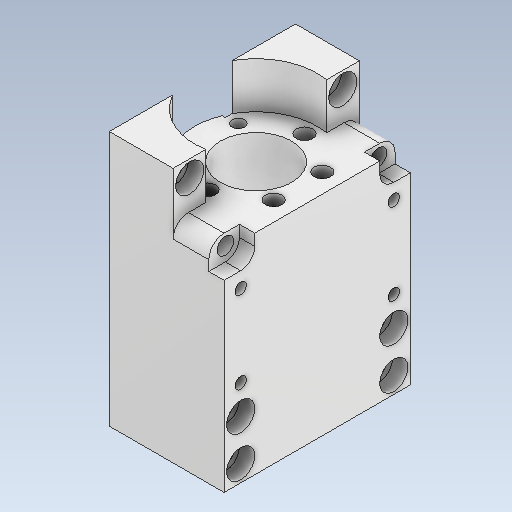
# Autodesk Inventor part: Z_carriage
Saved by Autodesk Inventor 2020 (Build 240168000, 168)
## iProperties
Created: 2022-03-20
Part Number: Z_carriage
Material: Tworzywo sztuczne ABS
Document SubType Name: Modeling
Designer: mikoma
Density: 1.06 g/cm^3
Appearance: Gładki — biały
Mass: 216.904 g
Surface Area: 569.885 cm^2
Volume: 204.626 cm^3
Author: mikoma
Autodesk Inventor part; units mm, degrees
ref_plane "YZ Plane" through (0, 0, 0) normal (1, 0, 0) x (0, 1, 0)
ref_plane "XZ Plane" through (0, 0, 0) normal (0, 1, 0) x (-1, 0, 0)
sketch "Szkic1" plane through (0, 0, 0) normal (1, 0, 0) x (0, 1, 0)
  line L0 (-50, 36.5) -> (50, 36.5)
  line L1 (50, 36.5) -> (50, -36.5)
  line L2 (50, -36.5) -> (-50, -36.5)
  line L3 (-50, -36.5) -> (-50, 36.5)
  line L4 (-50, 36.5) -> (50, -36.5) construction
  line L5 (50, 36.5) -> (-50, -36.5) construction
  point P0 (0, 0)
  dimension "d0" = 73
  dimension "d1" = 100
  constraints: 12 end point, 2 midpoint, 2 parallel, 1 horizontal, 1 perpendicular
  measures "d0" distance of L0.end L1.end
  measures "d1" distance of L1.end L2.end
extrude "Wyciągnięcie proste1" add sketch "Szkic1" along normal blind 45
sketch "Szkic2" plane through (0, 50, 36.5) normal (0, 1, 0) x (1, 0, 0)
  circle A0 centre (21, 36.5) radius 24
  line L0 (45, 73) -> (45, 0) projected
  line L1 (0, 73) -> (0, 0) projected
  circle A1 centre (21, 36.5) radius 14
  circle A2 centre (21, 36.5) radius 10
  point P0 (0, 36.5)
  point P1 (0, 36.5)
  dimension "d4" = 48
  dimension "d7" = 28
  dimension "d32" = 20
  constraints: 3 centre point, 2 coincident, 1 horizontal alignment, 1 midpoint, 1 tangent
  measures "d4" diameter of A0
  measures "d7" diameter of A1
  measures "d32" diameter of A2
extrude "Wyciągnięcie proste2" cut sketch "Szkic2" against normal blind 18 contours A0 L1 | L1 A0 | A1 | A2
sketch "Szkic3" plane through (0, -50, -36.5) normal (0, -1, 0) x (1, 0, 0)
  circle A0 centre (21, 36.5) radius 24
  arc A1 (0, 24.881) -> (45, 36.5) centre (21, 36.5) ccw projected
  line L0 (0, 73) -> (0, 0) projected
  line L1 (0, 27.5) -> (-1.2486, 27.5)
  line L2 (0, 45.5) -> (-1.2486, 45.5)
  line L3 (0, 27.5) -> (0, 45.5)
  dimension "d10" = 48
  dimension "d104" = 18
  dimension "d105" = 9
  constraints: 6 end point, 2 point on circle, 2 point on line, 1 centre point, 1 coincident, 1 collinear, 1 horizontal, 1 perpendicular
  measures "d10" diameter of A0
  measures "d104" distance between parallel lines of L2 L1
  measures "d105" distance from line of A0.centre L1
extrude "Wyciągnięcie proste4" add sketch "Szkic3" against normal up to surface (82 mm away) contours L2 L0 L1 A0
extrude "Wyciągnięcie proste5" cut sketch "Szkic2" against normal blind 44 contours A1 | A2
sketch "Szkic4" plane through (0, 0, 0) normal (-1, 0, 0) x (0, 0, 1)
  circle A0 centre (30, -43.5) radius 3.25
  line L0 (36.5, 50) -> (36.5, -50) projected
  line L1 (36.5, -50) -> (9, -50) projected
  circle A1 centre (30, -27.5) radius 3.25
  line L2 (0, 50) -> (0, 32) construction
  line L3 (0, 0) -> (0, 50)
  line L4 (0, 0) -> (36.5, 0) construction
  circle A2 centre (-30, -43.5) radius 3.25
  circle A3 centre (-30, -27.5) radius 3.25
  circle A4 centre (30, 43.5) radius 3.25
  circle A5 centre (30, 27.5) radius 3.25
  circle A6 centre (-30, 43.5) radius 3.25
  circle A7 centre (-30, 27.5) radius 3.25
  point P0 (11.619, -35)
  point P1 (-36.5, -50)
  dimension "d15" = 6.5
  dimension "d16" = 6.5
  dimension "d17" = 6.5
  dimension "d19" = 16
  constraints: 8 centre point, 7 symmetric about line, 4 end point, 1 equal radius, 1 midpoint, 1 vertical, 1 vertical alignment, 7 other
  measures "d15" diameter of A0
  measures "d16" distance from line of L0 A0.centre
  measures "d19" distance of A1.centre A0.centre
extrude "Wyciągnięcie proste6" cut sketch "Szkic4" against normal through all
sketch "Szkic5" plane through (0, 32, 36.5) normal (0, 1, 0) x (1, 0, 0)
  circle A0 centre (21, 55.5) radius 3.25
  circle A1 centre (21, 36.5) radius 14 projected
  circle A2 centre (21, 36.5) radius 19 construction
  circle A3 centre (37.4545, 46) radius 3.25
  circle A4 centre (37.4545, 27) radius 3.25
  circle A5 centre (21, 17.5) radius 3.25
  circle A6 centre (4.5455, 46) radius 2.5
  circle A7 centre (4.5455, 27) radius 2.5
  point P0 (0, 36.5)
  dimension "d22" = 6.5
  dimension "d23" = 38
  dimension "d83" = 180
  dimension "d95" = 5
  dimension "d96" = 5
  constraints: 7 centre point, 3 point on circle, 2 horizontal alignment, 1 coincident, 1 vertical alignment, 7 other
  measures "d22" diameter of A0
  measures "d23" diameter of A2
  measures "d95" diameter of A6
  measures "d96" diameter of A7
extrude "Wyciągnięcie proste7" cut sketch "Szkic5" against normal through all contours A0 | A3 | A4 | A5 | A6 | A7
sketch "Szkic6" plane through (45, 0, 0) normal (1, 0, 0) x (0, 0, -1)
  line L0 (-36.5, 50) -> (-36.5, -50) projected
  line L1 (-36.5, 50) -> (36.5, 50)
  line L2 (36.5, 50) -> (36.5, 32)
  line L3 (36.5, 32) -> (-36.5, 32)
  line L4 (-36.5, 32) -> (-36.5, 50)
  line L5 (15.75, 32) -> (22.25, 32) projected
  line L6 (-14, 32) -> (14, 32) projected
  line L7 (0, 32) -> (-11.619, 32) projected
  line L8 (11.619, 32) -> (0, 32) projected
  line L9 (-9, 32) -> (9, 32) projected
  line L10 (36.5, -50) -> (36.5, 50) projected
  line L11 (-11.619, 32) -> (-9, 32) projected
  line L12 (9, 32) -> (11.619, 32) projected
  point P0 (0, 0)
  point P1 (6.75, 17)
  point P2 (12.25, 17)
  point P3 (-12.25, 17)
  point P4 (-6.75, 17)
  point P5 (-12.25, 17)
  point P6 (-6.75, 17)
  point P7 (-21.75, 17)
  point P8 (-16.25, 17)
  point P9 (6.75, 17)
  point P10 (12.25, 17)
  point P11 (-36.5, 32)
  constraints: 8 end point, 2 parallel, 1 horizontal, 1 horizontal alignment, 1 perpendicular, 1 point on line
extrude "Wyciągnięcie proste8" cut sketch "Szkic6" against normal blind 20
extrude "Wyciągnięcie proste9" cut sketch "Szkic2" against normal through all contours A2
sketch "Szkic7" plane through (25, 0, 0) normal (1, 0, 0) x (0, 0, -1)
  circle A0 centre (-30, 43.5) radius 3.25 projected
  circle A1 centre (30, 43.5) radius 3.25 projected
  circle A2 centre (-30, 43.5) radius 5.5
  circle A3 centre (30, 43.5) radius 5.5
  point P0 (0, 0)
  dimension "d35" = 11
  dimension "d36" = 11
  constraints: 2 centre point, 2 coincident
  measures "d35" diameter of A2
  measures "d36" diameter of A3
extrude "Wyciągnięcie proste10" cut sketch "Szkic7" against normal blind 6 contours A0 | A1 | A2 | A3
sketch "Szkic8" plane through (45, 0, 0) normal (1, 0, 0) x (0, 0, -1)
  line L0 (36.5, -50) -> (36.5, 32) projected
  line L1 (-36.5, 32) -> (-36.5, -50) projected
  line L2 (-36.5, 16) -> (36.5, 16) construction
  line L3 (-36.5, -16) -> (36.5, -16) construction
  circle A0 centre (-30, 16) radius 2.25
  circle A1 centre (30, 16) radius 2.25
  circle A2 centre (-30, 27.5) radius 3.25 projected
  circle A3 centre (30, 27.5) radius 3.25 projected
  circle A4 centre (-30, -16) radius 2.25
  circle A5 centre (30, -16) radius 2.25
  circle A6 centre (-30, 16) radius 4
  circle A7 centre (-30, -16) radius 4
  circle A8 centre (30, -16) radius 4
  circle A9 centre (30, 16) radius 4
  line L4 (36.5, 32) -> (-36.5, 32) projected
  point P0 (0, 0)
  dimension "d44" = 32
  dimension "d47" = 4.5
  dimension "d53" = 8
  dimension "d54" = 8
  dimension "d55" = 8
  dimension "d56" = 8
  dimension "d71" = 16
  constraints: 8 centre point, 8 point on line, 4 coincident, 4 end point, 4 vertical alignment, 3 equal radius, 1 horizontal, 1 perpendicular
  measures "d44" distance between parallel lines of L3 L2
  measures "d47" diameter of A4
  measures "d53" diameter of A6
  measures "d54" diameter of A9
  measures "d55" diameter of A8
  measures "d56" diameter of A7
  measures "d71" distance from line of A9.centre L4
extrude "Wyciągnięcie proste11" cut sketch "Szkic8" against normal through all contours A0 | A1 | A4 | A5
ref_plane "Płaszczyzna konstrukcyjna1" through (35, 0, 0) normal (1, 0, 0) x (0, 0, -1)
extrude "Wyciągnięcie proste12" cut sketch "Szkic8" against normal up to surface (35 mm away) from surface at -10 contours A0 | A1 | A4 | A5 | A6 | A7 | A8 | A9
sketch "Szkic9" plane through (45, 0, 0) normal (1, 0, 0) x (0, 0, -1)
  circle A0 centre (-30, -27.5) radius 3.25 projected
  circle A1 centre (-30, -43.5) radius 3.25 projected
  circle A2 centre (30, -43.5) radius 3.25 projected
  circle A3 centre (30, -27.5) radius 3.25 projected
  circle A4 centre (30, 27.5) radius 3.25 projected
  circle A5 centre (-30, -27.5) radius 5.5
  circle A6 centre (-30, -43.5) radius 5.5
  circle A7 centre (30, -27.5) radius 3.25 projected
  circle A8 centre (30, -27.5) radius 5.5
  circle A9 centre (30, 27.5) radius 5.5
  circle A10 centre (30, -43.5) radius 5.5
  line L0 (30, 22) -> (36.5, 22)
  line L1 (24.5, 27.5) -> (24.5, 32)
  line L2 (26.8377, 32) -> (24.5, 32)
  circle A11 centre (-30, 27.5) radius 5.5
  line L3 (-36.5, 32) -> (-36.5, -50) projected
  line L4 (-36.5, 32) -> (-33.1623, 32)
  line L5 (-36.5, 22) -> (-30, 22)
  line L6 (-36.5, 32) -> (-36.5, 22)
  line L7 (-24.5, 27.5) -> (-24.5, 32)
  line L8 (-22.25, 32) -> (-15.75, 32) projected
  line L9 (-33.1623, 32) -> (-24.5, 32)
  line L10 (36.5, -50) -> (36.5, 50) projected
  line L11 (36.5, 32) -> (33.1623, 32)
  line L12 (36.5, 32) -> (36.5, 22)
  circle A12 centre (-30, 27.5) radius 3.25 projected
  point P0 (0, 0)
  point P1 (25.6689, 32)
  point P2 (-26.8377, 32)
  dimension "d106" = 11
  constraints: 20 end point, 8 point on circle, 7 coincident, 6 centre point, 5 equal radius, 4 horizontal, 4 tangent, 3 point on line, 2 horizontal alignment, 2 perpendicular, 2 vertical, 1 collinear, 1 midpoint, 1 parallel
  measures "d106" diameter of A11
extrude "Wyciągnięcie proste13" cut sketch "Szkic9" against normal blind 6 contours A0 | A1 | A2 | A3 | A4 | A5 | A6 | A8 | A9 | A9 L11 L10 L0 | A9 L1 L2 | A10 | L9 A11 | A11 L5 L3 L4 | A11 L9 | L9 L7 A11 | A12
sketch "Szkic10" plane through (0, -50, 36.5) normal (0, -1, 0) x (1, 0, 0)
  circle A0 centre (21, -36.5) radius 10 projected
  circle A1 centre (21, -55.5) radius 3.25 projected
  circle A2 centre (21, -17.5) radius 3.25 projected
  circle A3 centre (21, -36.5) radius 19 construction
  line L0 (24.1754, -61) -> (17.8246, -61)
  line L1 (17.8246, -61) -> (14.6491, -55.5)
  line L2 (14.6491, -55.5) -> (17.8246, -50)
  line L3 (17.8246, -50) -> (24.1754, -50)
  line L4 (24.1754, -50) -> (27.3509, -55.5)
  line L5 (27.3509, -55.5) -> (24.1754, -61)
  line L6 (34.2791, -40.5) -> (40.6299, -40.5)
  line L7 (31.1036, -46) -> (34.2791, -40.5)
  line L8 (34.2791, -51.5) -> (31.1036, -46)
  line L9 (40.6299, -51.5) -> (34.2791, -51.5)
  line L10 (43.8053, -46) -> (40.6299, -51.5)
  line L11 (40.6299, -40.5) -> (43.8053, -46)
  line L12 (31.1036, -27) -> (34.2791, -21.5)
  line L13 (34.2791, -32.5) -> (31.1036, -27)
  line L14 (40.6299, -32.5) -> (34.2791, -32.5)
  line L15 (43.8053, -27) -> (40.6299, -32.5)
  line L16 (40.6299, -21.5) -> (43.8053, -27)
  line L17 (34.2791, -21.5) -> (40.6299, -21.5)
  line L18 (17.8246, -23) -> (14.6491, -17.5)
  line L19 (24.1754, -23) -> (17.8246, -23)
  line L20 (27.3509, -17.5) -> (24.1754, -23)
  line L21 (24.1754, -12) -> (27.3509, -17.5)
  line L22 (17.8246, -12) -> (24.1754, -12)
  line L23 (14.6491, -17.5) -> (17.8246, -12)
  point P0 (21, -55.5)
  dimension "d97" = 11
  dimension "d100" = 180
  constraints: 48 end point, 2 coincident, 1 horizontal, 1 vertical alignment, 52 other
  measures "d97" distance between parallel lines of L1 L4
extrude "Wyciągnięcie proste14" cut sketch "Szkic10" against normal blind 45 contours A1 | A2 | L0 L1 L2 L3 L4 L5 | L6 L11 L10 L9 L8 L7 | L12 L17 L16 L15 L14 L13 | L18 L23 L22 L21 L20 L19
fillet "Zaokrąglenie1" radius 6 2 edges at (32, 32, 36.5) (32, 32, -36.5)
equation "\"d105\" = 0.5 * d104"
